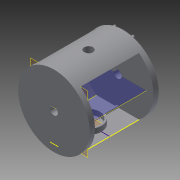
# Autodesk Inventor part: Fourth Diff
Saved by Autodesk Inventor 2015 (Build 190159000, 159)
## iProperties
Created: 2015-04-04
Part Number: Fourth Diff
Material: Generic
Document SubType Name: Modeling
Designer: Jack
Density: 1 g/cm^3
Appearance: Default
Author: Jack
Autodesk Inventor part; units mm, degrees
ref_plane "YZ Plane" through (0, 0, 0) normal (1, 0, 0) x (0, 1, 0)
ref_plane "XZ Plane" through (0, 0, 0) normal (0, 1, 0) x (-1, 0, 0)
ref_plane "XY Plane" through (0, 0, 0) normal (0, 0, 1) x (1, 0, 0)
sketch "Sketch1" plane through (0, 0, 0) normal (0, 0, 1) x (1, 0, 0)
  circle A0 centre (0, 0) radius 52.07
  dimension "d0" = 104.14
  constraints: 1 centre point, 1 coincident
  measures "d0" diameter of A0
extrude "Extrusion1" add sketch "Sketch1" along normal blind 7.62
ref_plane "Work Plane1" through (0, 0, 92.71) normal (0, 0, 1) x (1, 0, 0)
sketch "Sketch2" plane through (0, 0, 92.71) normal (0, 0, 1) x (1, 0, 0)
  circle A0 centre (0, 0) radius 52.07
  dimension "d4" = 104.14
  constraints: 1 centre point, 1 coincident
  measures "d4" diameter of A0
extrude "Extrusion2" add sketch "Sketch2" along normal blind 7.62
sketch "Sketch3" plane through (0, 0, 7.62) normal (0, 0, 1) x (1, 0, 0)
  circle A0 centre (0, 0) radius 52.07 projected
  line L0 (0, 52.07) -> (0, 41.91)
  line L1 (0, 41.91) -> (30.9004, 41.91)
  line L2 (0, 41.91) -> (-30.9004, 41.91)
  line L3 (0, 0) -> (20.3569, 0)
  dimension "d7" = 10.16
  constraints: 8 end point, 3 point on circle, 1 horizontal, 1 perpendicular, 1 point on line, 1 vertical
  measures "d7" distance of L0.start L0.end
ref_plane "Work Plane2" through (0, 0, 7.62) normal (0, -1, 0) x (1, 0, 0)
extrude "Extrusion3" add sketch "Sketch3" along normal blind 87.5665 contours L1 L0 A0 | A0 L0 L2
mirror "Mirror1" about plane through (0, 0, 7.62) normal (0, -1, 0) of "Extrusion3"
sketch "Sketch4" plane through (0, 0, 100.33) normal (0, 0, 1) x (1, 0, 0)
  circle A0 centre (0, 0) radius 5.715
  dimension "d11" = 11.43
  constraints: 1 centre point, 1 coincident
  measures "d11" diameter of A0
extrude "Extrusion4" cut sketch "Sketch4" against normal blind 101.6
sketch "Sketch5" plane through (0, 0, 7.62) normal (0, 0, 1) x (1, 0, 0)
  circle A0 centre (0, 0) radius 13.335
  circle A1 centre (0, 0) radius 5.715
  circle A2 centre (0, 0) radius 15.875
  dimension "d14" = 26.67
  dimension "d15" = 31.75
  constraints: 3 centre point, 3 coincident
  measures "d14" diameter of A0
  measures "d15" diameter of A2
extrude "Extrusion5" add sketch "Sketch5" along normal blind 7.62 contours A2
sketch "Sketch6" plane through (-30.9004, -41.91, 92.71) normal (0, 1, 0) x (1, 0, 0)
  line L0 (61.8009, 85.09) -> (61.8009, 0) projected
  line L1 (61.8009, 42.545) -> (33.4028, 42.545)
  line L2 (0, 85.09) -> (0, 0) projected
  line L3 (0, 42.545) -> (61.8009, 42.545)
  line L4 (36.6154, -7.62) -> (25.1854, -7.62) projected
  line L5 (30.9004, -7.62) -> (30.9004, 92.71)
  circle A0 centre (30.9004, 42.545) radius 6.35
  point P0 (61.8009, 0)
  point P1 (58.0758, -2.4765)
  dimension "d53" = 12.7
  constraints: 6 end point, 3 midpoint, 1 centre point, 1 collinear, 1 horizontal, 1 vertical, 2 other
  measures "d53" diameter of A0
extrude "Extrusion6" cut sketch "Sketch6" along normal mid plane 223.8375
sketch "Sketch10" plane through (0, 0, 0) normal (0, 0, -1) x (-1, 0, 0)
  circle A0 centre (0, 0) radius 5.715 projected
  line L0 (5.715, 0) -> (12.065, 0)
  line L1 (12.065, 0) -> (12.065, 50.6529)
  circle A1 centre (0, 0) radius 52.07 projected
  line L2 (12.065, 0) -> (12.065, -50.6529)
  line L3 (12.065, 0) -> (14.605, 0)
  line L4 (14.605, 0) -> (14.605, 49.9798)
  line L5 (14.605, 0) -> (14.605, -49.9798)
  line L6 (-5.715, 0) -> (-12.065, 0)
  line L7 (-12.065, 0) -> (-12.065, 50.6529)
  line L8 (-12.065, 0) -> (-12.065, -50.6529)
  line L9 (-12.065, 0) -> (-14.605, 0)
  line L10 (-14.605, 0) -> (-14.605, 49.9798)
  line L11 (-14.605, 0) -> (-14.605, -49.9798)
  dimension "d32" = 6.35
  dimension "d33" = 2.54
  dimension "d34" = 6.35
  dimension "d35" = 2.54
  constraints: 24 end point, 5 point on line, 4 perpendicular, 3 horizontal, 2 point on circle, 9 other
  measures "d32" distance of L0.start L0.end
  measures "d33" distance of L0.end L3.end
  measures "d34" distance of L6.start L6.end
  measures "d35" distance of L6.end L9.end
extrude "Extrusion10" add sketch "Sketch10" along normal blind 2.54 contours L3 L5 A1 L2 | L1 A1 L4 L3 | L9 L10 A1 L7 | L8 A1 L11 L9
sketch "Sketch14" plane through (0, 0, 0) normal (1, 0, 0) x (0, 1, 0)
  point P0 (0, 0)
sketch "Sketch15" plane through (-30.9004, -41.91, 7.62) normal (0, 1, 0) x (1, 0, 0)
  line L0 (61.8009, -85.09) -> (0, -85.09)
  line L1 (0, -85.09) -> (61.8009, -85.09) projected
  point P0 (30.9004, 7.62)
  point P1 (29.6304, -85.09)
  constraints: 2 end point, 1 collinear
ref_plane "Work Plane3" through (2.5024, -41.91, 50.165) normal (0, 1, 0) x (1, 0, 0)
sketch "Sketch18" plane through (-30.9004, -41.91, 7.62) normal (0, 1, 0) x (1, 0, 0)
  line L0 (61.8009, 0) -> (61.8009, -85.09) projected
  line L1 (61.8009, -42.545) -> (0, -42.545)
  line L2 (0, 0) -> (0, -85.09) projected
  line L3 (36.6154, -92.71) -> (25.1854, -92.71) projected
  line L4 (30.9004, -92.71) -> (30.9004, 7.62)
  constraints: 4 end point, 3 midpoint, 1 vertical
sketch "Sketch19" plane through (0, 0, 0) normal (1, 0, 0) x (0, 1, 0)
  line L0 (41.91, 7.62) -> (-41.91, 7.62) projected
  line L1 (27.4323, 7.62) -> (27.4323, 20.239)
  line L2 (27.4323, 20.239) -> (-18.8978, 20.239)
  line L3 (-18.8978, 20.239) -> (-18.8978, 7.62)
  line L4 (27.4323, 7.62) -> (-18.8978, 7.62)
  point P0 (0, 0)
  constraints: 8 end point, 2 perpendicular, 2 point on line, 1 collinear, 1 vertical
extrude "Extrusion16" cut sketch "Sketch19" along normal mid plane 101.6
sketch "Sketch20" plane through (-30.9004, 41.91, 7.62) normal (0, -1, 0) x (1, 0, 0)
  line L0 (0, 0) -> (0, 85.09) projected
  line L1 (0, 42.545) -> (61.8009, 42.545)
  line L2 (61.8009, 0) -> (61.8009, 85.09) projected
  circle A0 centre (30.9004, 42.545) radius 16.51
  circle A1 centre (30.9004, 42.545) radius 19.05
  point P0 (30.9004, -7.62)
  dimension "d61" = 33.02
  dimension "d62" = 38.1
  constraints: 3 midpoint, 2 centre point, 2 end point, 1 coincident
  measures "d61" diameter of A0
  measures "d62" diameter of A1
extrude "Extrusion17" add sketch "Sketch20" along normal blind 7.62 contours A0 L1 A1 | L1 A1 A0
mirror "Mirror3" about plane through (0, 0, 7.62) normal (0, -1, 0) of "Extrusion17"
sketch "Sketch21" plane through (-30.9004, -41.91, 92.71) normal (0, 1, 0) x (1, 0, 0)
  line L0 (0, 85.09) -> (61.8009, 85.09) projected
  line L1 (30.9004, 85.09) -> (32.1704, 85.09)
  line L2 (32.1704, 85.09) -> (30.9004, 85.09)
  line L3 (30.9004, 85.09) -> (29.6304, 85.09)
  line L4 (29.6304, 85.09) -> (29.6304, 61.5526)
  circle A0 centre (30.9004, 42.545) radius 19.05 projected
  line L5 (32.1704, 85.09) -> (32.1704, 61.5526)
  line L6 (29.6304, 61.5526) -> (32.1704, 61.5526)
  line L7 (61.8009, 0) -> (0, 0) projected
  line L8 (30.9004, 0) -> (29.6304, 0)
  line L9 (29.6304, 0) -> (32.1704, 0)
  line L10 (32.1704, 0) -> (32.1704, 23.5374)
  line L11 (29.6304, 0) -> (29.6304, 23.5374)
  line L12 (32.1704, 23.5374) -> (29.6304, 23.5374)
  point P0 (30.9004, 92.71)
  dimension "d65" = 1.27
  dimension "d66" = 1.27
  dimension "d67" = 1.27
  dimension "d68" = 1.27
  dimension "d69" = 2.54
  constraints: 22 end point, 4 point on circle, 4 point on line, 3 perpendicular, 2 midpoint, 1 collinear, 1 parallel
  measures "d65" distance of L1.start L1.end
  measures "d66" distance of L1.end L1.start
  measures "d67" distance of L1.start L3.end
  measures "d68" distance of L8.start L8.end
  measures "d69" distance of L8.end L9.end
extrude "Extrusion18" add sketch "Sketch21" along normal blind 2.54 contours L0 L5 A0 L4 | A0 L10 L7 L11
mirror "Mirror4" about plane through (0, 0, 7.62) normal (0, -1, 0) of "Extrusion18"
body "Solid1"
